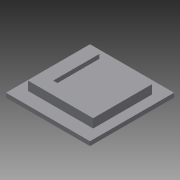
# Autodesk Inventor part: SpoolHolderSplitBase
Saved by Autodesk Inventor 2015 SP1 (Build 190203100, 203)
## iProperties
Created: 2015-04-19
Part Number: SpoolHolderSplitBase
Material: Generic
Document SubType Name: Modeling
Designer: Jack
Density: 1 g/cm^3
Appearance: Default
Author: Jack
Autodesk Inventor part; units mm, degrees
ref_plane "YZ Plane" through (0, 0, 0) normal (1, 0, 0) x (0, 1, 0)
ref_plane "XZ Plane" through (0, 0, 0) normal (0, 1, 0) x (-1, 0, 0)
ref_plane "XY Plane" through (0, 0, 0) normal (0, 0, 1) x (1, 0, 0)
sketch "Sketch1" plane through (0, 0, 0) normal (0, 0, 1) x (1, 0, 0)
  line L0 (0, 0) -> (80, 0)
  line L1 (80, 0) -> (80, 80)
  line L2 (80, 80) -> (0, 80)
  line L3 (0, 80) -> (0, 0)
  dimension "d0" = 80
  dimension "d1" = 80
  constraints: 8 end point, 2 parallel, 1 horizontal, 1 perpendicular
  measures "d0" distance of L2.end L1.end
  measures "d1" distance of L1.end L0.end
extrude "Extrusion1" add sketch "Sketch1" along normal blind 4
sketch "Sketch2" plane through (0, 0, 4) normal (0, 0, 1) x (1, 0, 0)
  line L0 (0, 0) -> (80, 0) projected
  line L1 (80, 0) -> (80, 80) projected
  line L2 (9, 68) -> (9, 12)
  line L3 (9, 12) -> (71, 12)
  line L4 (71, 12) -> (71, 68)
  line L5 (71, 68) -> (65, 68)
  line L6 (65, 68) -> (65, 18)
  line L7 (65, 18) -> (15, 18)
  line L8 (15, 18) -> (15, 68)
  line L9 (15, 68) -> (9, 68)
  dimension "d4" = 6
  dimension "d5" = 6
  dimension "d6" = 50
  dimension "d7" = 50
  dimension "d8" = 9
  dimension "d9" = 12
  constraints: 16 end point, 7 perpendicular, 1 collinear, 1 point on line, 1 vertical
  measures "d4" distance of L4.end L5.end
  measures "d5" distance between parallel lines of L3 L7
  measures "d6" distance of L6.end L7.end
  measures "d7" distance of L7.end L8.end
  measures "d8" distance between parallel lines of L1 L4
  measures "d9" distance between parallel lines of L0 L3
extrude "Extrusion2" add sketch "Sketch2" along normal blind 4.5
sketch "Sketch3" plane through (0, 0, 8.5) normal (0, 0, 1) x (1, 0, 0)
  line L0 (9, 68) -> (9, 12) projected
  line L1 (9, 12) -> (71, 12) projected
  line L2 (71, 12) -> (71, 68) projected
  line L3 (71, 68) -> (65, 68) projected
  line L4 (65, 68) -> (65, 18) projected
  line L5 (65, 18) -> (15, 18) projected
  line L6 (15, 18) -> (15, 68) projected
  line L7 (15, 68) -> (9, 68) projected
  line L8 (15, 68) -> (21, 68)
  line L9 (21, 68) -> (21, 24)
  line L10 (21, 24) -> (59, 24)
  line L11 (59, 24) -> (59, 68)
  line L12 (59, 68) -> (65, 68)
  point P0 (0, 0)
  dimension "d12" = 6
  dimension "d13" = 6
  constraints: 10 end point, 4 perpendicular, 1 collinear, 1 horizontal, 1 point on line
  measures "d12" distance of L6.end L8.end
  measures "d13" distance between parallel lines of L5 L10
extrude "Extrusion3" add sketch "Sketch3" along normal blind 4
body "Solid1"
